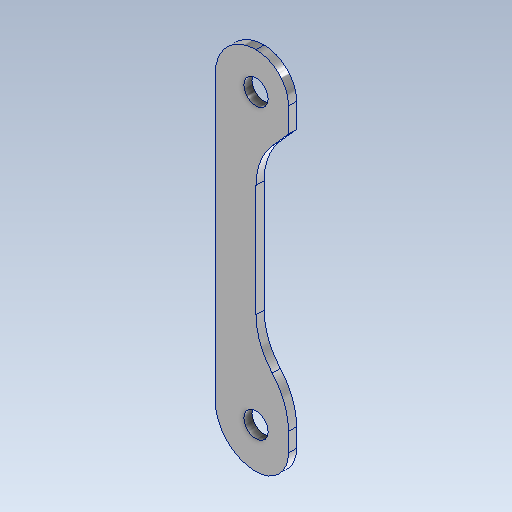
# Autodesk Inventor part: arm1b
Saved by Autodesk Inventor 2020.3 (Build 243373000, 373)
## iProperties
Created: 2016-01-12
Part Number: arm1b
Material: Aluminum 6061
Document SubType Name: Modeling
Designer: Nanjar
Density: 2.7 g/cm^3
Appearance: Aluminum - Flat
Author: Nanjar
Autodesk Inventor part; units mm, degrees
ref_plane "YZ Plane" through (0, 0, 0) normal (1, 0, 0) x (0, 1, 0)
ref_plane "XZ Plane" through (0, 0, 0) normal (0, 1, 0) x (-1, 0, 0)
ref_plane "XY Plane" through (0, 0, 0) normal (0, 0, 1) x (1, 0, 0)
sketch "Sketch3" plane through (0, 0, 0) normal (0, 0, 1) x (1, 0, 0)
  circle A0 centre (0, 0) radius 1.5
  circle A1 centre (0, 35.5) radius 1.5
  line L0 (0, 8.5) -> (4, 4.5)
  line L1 (4, 40) -> (4, 33)
  line L2 (4, 4.5) -> (4, -5)
  line L3 (4, 40) -> (-5, 40)
  line L4 (4, -5) -> (-5, -5)
  line L5 (-5, 40) -> (-5, -5)
  line L6 (4, 33) -> (4, 33.5)
  line L7 (4, 33) -> (0, 28.5)
  line L8 (0, 28.5) -> (0, 35.5) construction
  line L9 (0, 8.5) -> (0, 0) construction
  line L10 (0, 0) -> (0, -5) construction
  line L11 (0, 28.5) -> (0, 8.5)
  dimension "d27" = 45
  dimension "d28" = 4.5
  dimension "d34" = 7
  constraints: 24 end point, 3 vertical, 2 centre point, 2 point on line, 1 coincident, 1 perpendicular
  measures "d27" distance between parallel lines of L4 L3
  measures "d28" distance from line of L8.end L3
  measures "d34" distance of L7.end L8.end
extrude "Extrusion2" add sketch "Sketch3" along normal blind 1
fillet "Fillet4" radius 4 2 edges at (4, 40, 0.5) (4, -5, 0.5)
fillet "Fillet6" radius 5 2 edges at (-5, 40, 0.5) (-5, -5, 0.5)
fillet "Fillet7" radius 7.8 3 edges at (0, 28.5, 0.5) (0, 8.5, 0.5) (4, 4.5, 0.5)
body "Solid2"
